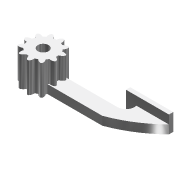
# Autodesk Inventor part: Greifer2
Saved by Autodesk Inventor 2015 (Build 190159000, 159)
## iProperties
Created: 2015-02-07
Part Number: Greifer2
Material: ABS-Kunststoff
Document SubType Name: Modeling
Designer: Luki
Density: 1.06 g/cm^3
Appearance: Chrom - poliert
Author: Luki
Autodesk Inventor part; units mm, degrees
ref_plane "YZ Plane" through (0, 0, 0) normal (1, 0, 0) x (0, 1, 0)
ref_plane "XZ Plane" through (0, 0, 0) normal (0, 1, 0) x (-1, 0, 0)
ref_plane "XY Plane" through (0, 0, 0) normal (0, 0, 1) x (1, 0, 0)
sketch "Skizze1" plane through (0, 0, 0) normal (0, 0, 1) x (1, 0, 0)
  circle A0 centre (0, 0) radius 7.5
  circle A1 centre (0, 0) radius 2
  circle A2 centre (0, 0) radius 6.5
  circle A3 centre (0, 0) radius 8.5
  line L0 (0, 11.9067) -> (0, -11.9011) projected
  line L1 (-11.9, 0) -> (11.9, 0) projected
  line L2 (0, 0) -> (2.2933, 8.1848)
  line L3 (0, 0) -> (4.4165, 7.2626)
  arc A4 (0, 7.5) -> (-0.3402, 6.4911) centre (2.4347, 6.1172) ccw
  arc A5 (0.8885, 8.4534) -> (0, 7.5) centre (2.4473, 6.1101) ccw
  arc A6 (2.0235, 7.2219) -> (1.4252, 8.3797) centre (-0.708, 6.5438) ccw
  arc A7 (2.0788, 6.1586) -> (2.0235, 7.2219) centre (-0.694, 6.5473) ccw
  line L4 (0, 0) -> (-0.3402, 6.4911)
  line L5 (0, 0) -> (2.0788, 6.1586)
  line L6 (0.8885, 8.4534) -> (0, 0)
  line L7 (0, 0) -> (1.4252, 8.3797)
  arc A8 (0, 7.5) -> (-0.3402, 6.4911) centre (2.4347, 6.1172) ccw
  arc A9 (0.8885, 8.4534) -> (0, 7.5) centre (2.4473, 6.1101) ccw
  arc A10 (2.0235, 7.2219) -> (1.4252, 8.3797) centre (-0.708, 6.5438) ccw
  arc A11 (2.0788, 6.1586) -> (2.0235, 7.2219) centre (-0.694, 6.5473) ccw
  arc A12 (2.0788, 6.1586) -> (-0.3402, 6.4911) centre (0, 0) ccw
  dimension "d0" = 15
  dimension "d1" = 4
  dimension "d2" = 1
  dimension "d3" = 1
  dimension "d4" = 15.652
  dimension "d5" = 15.652
  dimension "d6" = 3
  dimension "d7" = 3
  dimension "d9" = 6
  dimension "d10" = 6
  dimension "d11" = 2.8
  dimension "d12" = 2.8
  constraints: 26 point on circle, 13 centre point, 12 end point, 7 tangent, 4 coincident, 3 concentric, 2 point on line
  measures "d0" diameter of A0
  measures "d1" diameter of A1
  measures "d2" radial gap between concentric circles of A0 A2
  measures "d3" radial gap between concentric circles of A3 A0
  measures "d4" angle of L0 L2
  measures "d5" angle of L2 L3
  measures "d6" angle of L0 L4
  measures "d7" angle of L2 L5
  measures "d9" angle of L0 L6
  measures "d10" angle of L2 L7
  measures "d11" radius of A4
  measures "d12" radius of A7
extrude "Extrusion1" add sketch "Skizze1" along normal blind 14 contours L2 A2 L7 A0 | A7 A2 L2 | A0 L7 A6 | L7 A2 L6 A0 | A0 L6 A3 L7 | L2 A1 L7 A2 | A5 L6 A0 | A0 L6 A2 L0 | L0 A2 A4 | L4 A1 L0 | L7 A1 L2 | L0 A1 L6 | L6 A1 L7 | L7 A1 L6 A2 | L0 A1 L4 A2 | A2 L6 A1 L0
pattern_circular "Runde Anordnung1" count 11 over 360 about axis through (0, 0, -10) along (0, 0, 1) of "Extrusion1"
sketch "Skizze2" plane through (0, 0, 14) normal (0, 0, 1) x (0.8118, 0.5839, 0)
  arc A0 (5.6575, 6.3437) -> (4.3795, 6.0885) centre (5.5546, 3.5312) ccw projected
  arc A1 (6.0501, 5.9705) -> (5.6575, 6.3437) centre (0, 0) ccw projected
  arc A2 (5.8597, 4.6812) -> (6.0501, 5.9705) centre (3.2463, 5.7257) ccw projected
  arc A3 (5.2838, 3.7857) -> (5.8597, 4.6812) centre (3.2597, 5.7204) ccw projected
  arc A4 (5.2838, 3.7857) -> (5.0784, 4.057) centre (0, 0) ccw projected
  line L0 (5.0784, 4.057) -> (0, 0) projected
  line L1 (0, 0) -> (5.9126, 2.7002) projected
  arc A5 (6.9759, 2.7543) -> (5.9126, 2.7002) centre (6.5839, -0.0181) ccw projected
  arc A6 (8.1891, 2.278) -> (6.9759, 2.7543) centre (6.5819, -0.0324) ccw projected
  arc A7 (8.3175, 1.7518) -> (8.1891, 2.278) centre (0, 0) ccw projected
  arc A8 (7.4604, 0.7701) -> (8.3175, 1.7518) centre (5.8266, 3.0617) ccw projected
  arc A9 (6.4917, 0.3281) -> (7.4604, 0.7701) centre (5.8349, 3.05) ccw projected
  arc A10 (6.4917, 0.3281) -> (6.4656, 0.6674) centre (0, 0) ccw projected
  line L2 (6.4656, 0.6674) -> (0, 0) projected
  line L3 (0, 0) -> (-4.9124, -4.2566) projected
  arc A11 (-5.9174, -4.6081) -> (-4.9124, -4.2566) centre (-6.3224, -1.8375) ccw projected
  arc A12 (-7.2155, -4.4929) -> (-5.9174, -4.6081) centre (-6.3244, -1.8233) ccw projected
  arc A13 (-7.4871, -4.0241) -> (-7.2155, -4.4929) centre (0, 0) ccw projected
  arc A14 (-6.9412, -2.8407) -> (-7.4871, -4.0241) centre (-4.728, -4.5792) ccw projected
  arc A15 (-6.1363, -2.1437) -> (-6.9412, -2.8407) centre (-4.7393, -4.5703) ccw projected
  arc A16 (-6.1363, -2.1437) -> (-6.0157, -2.4619) centre (0, 0) ccw projected
  line L4 (-6.0157, -2.4619) -> (0, 0) projected
  line L5 (-6.3918, 1.1812) -> (0, 0) projected
  arc A17 (-6.3212, 1.5141) -> (-6.3918, 1.1812) centre (0, 0) ccw projected
  arc A18 (-6.3212, 1.5141) -> (-7.3751, 1.363) centre (-6.4578, -1.2825) ccw projected
  arc A19 (-7.3751, 1.363) -> (-8.4741, 0.6625) centre (-6.4531, -1.2961) ccw projected
  arc A20 (-8.4741, 0.6625) -> (-8.4991, 0.1214) centre (0, 0) ccw projected
  arc A21 (-8.4991, 0.1214) -> (-7.4693, -0.6774) centre (-6.3062, 1.8854) ccw projected
  arc A22 (-7.4693, -0.6774) -> (-6.4338, -0.925) centre (-6.3121, 1.8723) ccw projected
  line L6 (0, 0) -> (-6.4338, -0.925) projected
  line L7 (-3.7297, -5.3235) -> (0, 0) projected
  arc A23 (-4.0032, -5.121) -> (-3.7297, -5.3235) centre (0, 0) ccw projected
  arc A24 (-4.0032, -5.121) -> (-4.3035, -6.1425) centre (-1.516, -6.4071) ccw projected
  arc A25 (-4.3035, -6.1425) -> (-4.1229, -7.4331) centre (-1.5017, -6.4084) ccw projected
  arc A26 (-4.1229, -7.4331) -> (-3.6411, -7.6807) centre (0, 0) ccw projected
  arc A27 (-3.6411, -7.6807) -> (-2.4867, -7.0757) centre (-4.3347, -4.9531) ccw projected
  arc A28 (-2.4867, -7.0757) -> (-1.8313, -6.2367) centre (-4.3253, -4.9639) ccw projected
  line L8 (0, 0) -> (-1.8313, -6.2367) projected
  arc A29 (4.3795, 6.0885) -> (3.5142, 5.4681) centre (5.5486, 3.5443) ccw projected
  line L9 (0, 0) -> (3.5142, 5.4681) projected
  line L10 (-4.7385, 4.4494) -> (0, 0) projected
  line L11 (0, 0) -> (1.8313, -6.2367) projected
  arc A30 (1.7335, -7.2969) -> (1.8313, -6.2367) centre (-0.9549, -6.5144) ccw projected
  arc A31 (1.0894, -8.4299) -> (1.7335, -7.2969) centre (-0.9688, -6.5103) ccw projected
  arc A32 (0.5502, -8.4822) -> (1.0894, -8.4299) centre (0, 0) ccw projected
  arc A33 (-0.2995, -7.494) -> (0.5502, -8.4822) centre (2.2013, -6.203) ccw projected
  arc A34 (-0.5991, -6.4723) -> (-0.2995, -7.494) centre (2.1885, -6.2096) ccw projected
  arc A35 (-0.5991, -6.4723) -> (-0.2596, -6.4948) centre (0, 0) ccw projected
  line L12 (-0.2596, -6.4948) -> (0, 0) projected
  line L13 (-1.5808, 6.3049) -> (0, 0) projected
  arc A36 (-1.2486, 6.3789) -> (-1.5808, 6.3049) centre (0, 0) ccw projected
  arc A37 (-1.2486, 6.3789) -> (-1.824, 7.2748) centre (-3.8493, 5.3415) ccw projected
  arc A38 (-1.824, 7.2748) -> (-2.9176, 7.9836) centre (-3.8597, 5.3315) ccw projected
  arc A39 (-2.9176, 7.9836) -> (-3.4203, 7.7815) centre (0, 0) ccw projected
  arc A40 (-3.4203, 7.7815) -> (-3.719, 6.513) centre (-0.9047, 6.5195) ccw projected
  arc A41 (-3.719, 6.513) -> (-3.5142, 5.4681) centre (-0.919, 6.5195) ccw projected
  line L14 (0, 0) -> (-3.5142, 5.4681) projected
  line L15 (3.293, -5.6041) -> (0, 0) projected
  arc A42 (2.9952, -5.7688) -> (3.293, -5.6041) centre (0, 0) ccw projected
  arc A43 (2.9952, -5.7688) -> (3.7996, -6.4663) centre (5.1983, -4.0406) ccw projected
  arc A44 (3.7996, -6.4663) -> (5.0487, -6.8382) centre (5.2055, -4.0282) ccw projected
  arc A45 (5.0487, -6.8382) -> (5.474, -6.5027) centre (0, 0) ccw projected
  arc A46 (5.474, -6.5027) -> (5.4033, -5.2014) centre (2.7048, -6.0006) ccw projected
  arc A47 (5.4033, -5.2014) -> (4.9124, -4.2566) centre (2.7186, -5.9965) ccw projected
  line L16 (0, 0) -> (4.9124, -4.2566) projected
  arc A48 (-4.4991, 4.6913) -> (-4.7385, 4.4494) centre (0, 0) ccw projected
  arc A49 (-4.4991, 4.6913) -> (-5.4675, 5.1339) centre (-6.1261, 2.4124) ccw projected
  arc A50 (-5.4675, 5.1339) -> (-6.7707, 5.1388) centre (-6.1295, 2.3984) ccw projected
  arc A51 (-6.7707, 5.1388) -> (-7.0843, 4.6971) centre (0, 0) ccw projected
  arc A52 (-7.0843, 4.6971) -> (-6.6498, 3.4684) centre (-4.2858, 4.9955) ccw projected
  arc A53 (-6.6498, 3.4684) -> (-5.9126, 2.7002) centre (-4.2979, 4.9877) ccw projected
  line L17 (0, 0) -> (-5.9126, 2.7002) projected
  line L18 (2.0788, 6.1586) -> (0, 0) projected
  line L19 (0, 0) -> (6.4338, -0.925) projected
  arc A54 (7.3576, -1.4544) -> (6.4338, -0.925) centre (5.529, -3.5748) ccw projected
  arc A55 (8.1207, -2.5109) -> (7.3576, -1.4544) centre (5.5196, -3.5857) ccw projected
  arc A56 (7.9442, -3.0231) -> (8.1207, -2.5109) centre (0, 0) ccw projected
  arc A57 (6.6924, -3.3856) -> (7.9442, -3.0231) centre (6.5569, -0.5744) ccw projected
  arc A58 (5.6386, -3.2337) -> (6.6924, -3.3856) centre (6.5576, -0.5888) ccw projected
  arc A59 (5.6386, -3.2337) -> (5.8001, -2.9341) centre (0, 0) ccw projected
  line L20 (5.8001, -2.9341) -> (0, 0) projected
  arc A60 (2.3983, 6.0414) -> (2.0788, 6.1586) centre (0, 0) ccw projected
  arc A61 (2.3983, 6.0414) -> (2.3987, 7.1061) centre (-0.3504, 6.5746) ccw projected
  arc A62 (2.3987, 7.1061) -> (1.8618, 8.2936) centre (-0.3646, 6.5719) ccw projected
  arc A63 (1.8618, 8.2936) -> (1.3297, 8.3954) centre (0, 0) ccw projected
  arc A64 (1.3297, 8.3954) -> (0.3925, 7.4897) centre (2.7637, 5.9737) ccw projected
  arc A65 (0.3925, 7.4897) -> (0, 6.5) centre (2.7516, 5.9814) ccw projected
  line L21 (0, 0) -> (0, 6.5) projected
  circle A66 centre (0, 0) radius 6.5
  constraints: 1 centre point, 1 coincident
extrude "Extrusion2" add sketch "Skizze2" against normal blind 14 contours A66 L0 L9 | L9 L18 A60 A66 | L0 A4 A66 L1 | L1 A66 L2 | L7 A23 A66 L3 | L3 A66 L4 | L6 A66 L5 | L4 A16 A66 L6 | L8 A66 L7 | L12 A35 A66 L8 | L17 A66 L10 | L15 A42 A66 L11 | L11 A66 L12 | L14 A66 L13 | L10 A48 A66 L14 | L16 A66 L15 | L20 A59 A66 L16 | L5 A17 A66 L17 | L21 A66 L18 | L2 A10 A66 L19 | L19 A66 L20 | L13 A36 A66 L21
sketch "Skizze3" plane through (0, 0, 0) normal (0, 0, -1) x (-1, 0, 0)
  line L0 (0, -19.7919) -> (0, 59.2516) projected
  line L1 (-62.4254, 0) -> (20.3695, 0) projected
  arc A0 (0, 7.5) -> (-0.8885, 8.4534) centre (-2.4473, 6.1101) ccw projected
  arc A1 (0.3402, 6.4911) -> (0, 7.5) centre (-2.4347, 6.1172) ccw projected
  arc A2 (1.5808, 6.3049) -> (0.3402, 6.4911) centre (0, 0) ccw projected
  arc A3 (2.2022, 7.1694) -> (1.5808, 6.3049) centre (4.1236, 5.1327) ccw projected
  arc A4 (3.3315, 7.8199) -> (2.2022, 7.1694) centre (4.1335, 5.1222) ccw projected
  arc A5 (3.8228, 7.5918) -> (3.3315, 7.8199) centre (0, 0) ccw projected
  arc A6 (4.0548, 6.3094) -> (3.8228, 7.5918) centre (1.2446, 6.4633) ccw projected
  arc A7 (3.7955, 5.2767) -> (4.0548, 6.3094) centre (1.259, 6.4625) ccw projected
  arc A8 (4.7385, 4.4494) -> (3.7955, 5.2767) centre (0, 0) ccw projected
  arc A9 (5.7287, 4.8407) -> (4.7385, 4.4494) centre (6.2439, 2.0885) ccw projected
  arc A10 (7.0304, 4.7774) -> (5.7287, 4.8407) centre (6.2466, 2.0744) ccw projected
  arc A11 (7.3204, 4.3199) -> (7.0304, 4.7774) centre (0, 0) ccw projected
  arc A12 (6.8222, 3.1156) -> (7.3204, 4.3199) centre (4.5413, 4.7644) ccw projected
  arc A13 (6.0458, 2.3871) -> (6.8222, 3.1156) centre (4.553, 4.7559) ccw projected
  arc A14 (6.3918, 1.1812) -> (6.0458, 2.3871) centre (0, 0) ccw projected
  arc A15 (7.4363, 0.9751) -> (6.3918, 1.1812) centre (6.3819, -1.6188) ccw projected
  arc A16 (8.4972, 0.2181) -> (7.4363, 0.9751) centre (6.3765, -1.6321) ccw projected
  arc A17 (8.4938, -0.3236) -> (8.4972, 0.2181) centre (0, 0) ccw projected
  arc A18 (7.4237, -1.0674) -> (8.4938, -0.3236) centre (6.3962, 1.5528) ccw projected
  arc A19 (6.3766, -1.2605) -> (7.4237, -1.0674) centre (6.4015, 1.5394) ccw projected
  arc A20 (6.0157, -2.4619) -> (6.3766, -1.2605) centre (0, 0) ccw projected
  arc A21 (6.783, -3.2001) -> (6.0157, -2.4619) centre (4.4936, -4.8121) ccw projected
  arc A22 (7.2662, -4.4104) -> (6.783, -3.2001) centre (4.4818, -4.8204) ccw projected
  arc A23 (6.9705, -4.8643) -> (7.2662, -4.4104) centre (0, 0) ccw projected
  arc A24 (5.6681, -4.9115) -> (6.9705, -4.8643) centre (6.2204, -2.1518) ccw projected
  arc A25 (4.6829, -4.5079) -> (5.6681, -4.9115) centre (6.2175, -2.1659) ccw projected
  arc A26 (3.7297, -5.3235) -> (4.6829, -4.5079) centre (0, 0) ccw projected
  arc A27 (3.9761, -6.3593) -> (3.7297, -5.3235) centre (1.1787, -6.4776) ccw projected
  arc A28 (3.7283, -7.6387) -> (3.9761, -6.3593) centre (1.1643, -6.4782) ccw projected
  arc A29 (3.2341, -7.8607) -> (3.7283, -7.6387) centre (0, 0) ccw projected
  arc A30 (2.113, -7.1962) -> (3.2341, -7.8607) centre (4.0696, -5.1732) ccw projected
  arc A31 (1.5023, -6.324) -> (2.113, -7.1962) centre (4.0595, -5.1835) ccw projected
  arc A32 (0.2596, -6.4948) -> (1.5023, -6.324) centre (0, 0) ccw projected
  arc A33 (-0.0931, -7.4994) -> (0.2596, -6.4948) centre (-2.5105, -6.0865) ccw projected
  arc A34 (-0.9934, -8.4418) -> (-0.0931, -7.4994) centre (-2.5229, -6.0793) ccw projected
  arc A35 (-1.5291, -8.3613) -> (-0.9934, -8.4418) centre (0, 0) ccw projected
  arc A36 (-2.113, -7.1962) -> (-1.5291, -8.3613) centre (0.6267, -6.5521) ccw projected
  arc A37 (-2.1552, -6.1323) -> (-2.113, -7.1962) centre (0.6127, -6.5554) ccw projected
  arc A38 (-3.293, -5.6041) -> (-2.1552, -6.1323) centre (0, 0) ccw projected
  arc A39 (-4.1328, -6.2586) -> (-3.293, -5.6041) centre (-5.4026, -3.763) ccw projected
  arc A40 (-5.3996, -6.5646) -> (-4.1328, -6.2586) centre (-5.4091, -3.7502) ccw projected
  arc A41 (-5.8068, -6.2073) -> (-5.3996, -6.5646) centre (0, 0) ccw projected
  arc A42 (-5.6681, -4.9115) -> (-5.8068, -6.2073) centre (-3.0151, -5.8508) ccw projected
  arc A43 (-5.1284, -3.9937) -> (-5.6681, -4.9115) centre (-3.0287, -5.846) ccw projected
  arc A44 (-5.8001, -2.9341) -> (-5.1284, -3.9937) centre (0, 0) ccw projected
  arc A45 (-6.8604, -3.0307) -> (-5.8001, -2.9341) centre (-6.5794, -0.2448) ccw projected
  arc A46 (-8.0916, -2.6032) -> (-6.8604, -3.0307) centre (-6.578, -0.2305) ccw projected
  arc A47 (-8.2409, -2.0825) -> (-8.0916, -2.6032) centre (0, 0) ccw projected
  arc A48 (-7.4237, -1.0674) -> (-8.2409, -2.0825) centre (-5.6997, -3.2919) ccw projected
  arc A49 (-6.4734, -0.5871) -> (-7.4237, -1.0674) centre (-5.7085, -3.2805) ccw projected
  arc A50 (-6.4656, 0.6674) -> (-6.4734, -0.5871) centre (0, 0) ccw projected
  arc A51 (-7.4098, 1.1595) -> (-6.4656, 0.6674) centre (-5.6673, 3.3512) ccw projected
  arc A52 (-8.2145, 2.1847) -> (-7.4098, 1.1595) centre (-5.6583, 3.3624) ccw projected
  arc A53 (-8.0586, 2.7035) -> (-8.2145, 2.1847) centre (0, 0) ccw projected
  arc A54 (-6.8222, 3.1156) -> (-8.0586, 2.7035) centre (-6.5746, 0.3121) ccw projected
  arc A55 (-5.7632, 3.0059) -> (-6.8222, 3.1156) centre (-6.5759, 0.3265) ccw projected
  arc A56 (-5.0784, 4.057) -> (-5.7632, 3.0059) centre (0, 0) ccw projected
  arc A57 (-5.6067, 4.9815) -> (-5.0784, 4.057) centre (-2.9559, 5.8832) ccw projected
  arc A58 (-5.7293, 6.2789) -> (-5.6067, 4.9815) centre (-2.9422, 5.8878) ccw projected
  arc A59 (-5.3177, 6.6311) -> (-5.7293, 6.2789) centre (0, 0) ccw projected
  arc A60 (-4.0548, 6.3094) -> (-5.3177, 6.6311) centre (-5.3622, 3.8171) ccw projected
  arc A61 (-3.2232, 5.6446) -> (-4.0548, 6.3094) centre (-5.3555, 3.8298) ccw projected
  arc A62 (-2.0788, 6.1586) -> (-3.2232, 5.6446) centre (0, 0) ccw projected
  arc A63 (-2.0235, 7.2219) -> (-2.0788, 6.1586) centre (0.694, 6.5473) ccw projected
  arc A64 (-1.4252, 8.3797) -> (-2.0235, 7.2219) centre (0.708, 6.5438) ccw projected
  arc A65 (-0.8885, 8.4534) -> (-1.4252, 8.3797) centre (0, 0) ccw projected
  circle A66 centre (0, 0) radius 3.5
  line L2 (-50, 10.5) -> (-30, 10.5)
  line L3 (-30, 10.5) -> (-30, 8.5)
  line L4 (-30, 8.5) -> (-50, 8.5)
  line L5 (-50, 8.5) -> (-50, 10.5)
  circle A67 centre (0, 0) radius 8.5
  arc A68 (-5.3177, 6.6311) -> (-5.7293, 6.2789) centre (0, 0) ccw projected
  line L6 (0, -3.5) -> (-31, -3.5)
  line L7 (-31, -3.5) -> (-31, 3.5)
  line L8 (-31, 3.5) -> (0, 3.5)
  line L9 (0, 3.5) -> (0, -3.5)
  arc A69 (-34.873, 8.5) -> (-31, 3.5) centre (-31, 7.5) ccw
  arc A70 (-50, 8.5) -> (-31, -3.5) centre (-12.2955, 47.1571) ccw
  dimension "d24" = 7
  dimension "d20" = 2
  dimension "d21" = 0
  dimension "d22" = 50
  dimension "d23" = 30
  dimension "d25" = 54
  dimension "d26" = 7
  dimension "d27" = 4
  dimension "d28" = 31
  constraints: 16 end point, 4 parallel, 4 point on circle, 3 centre point, 2 coincident, 2 horizontal, 2 perpendicular, 2 point on line, 2 tangent, 1 vertical alignment, 2 other
  measures "d20" distance between parallel lines of L2 L4
  measures "d21" distance edge to line of A67 L4
  measures "d22" distance between parallel lines of L0 L5
  measures "d23" distance between parallel lines of L0 L3
  measures "d25" radius of A70
  measures "d26" distance from line of L8 L6.end
  measures "d27" radius of A69
  measures "d28" distance between parallel lines of L0 L7
extrude "Extrusion3" add sketch "Skizze3" against normal blind 4 contours A66 L1 L0 | L0 L1 A66 | A66 L1 A50 A51 A52 A53 A54 A55 A56 L8 | L1 A66 L0 | L0 A66 L1 | A66 L6 A44 A45 A46 A47 A48 A49 A50 L1 | A56 A55 A54 A67 L8 | A50 A49 A48 A67 L1 | L1 A67 A52 A51 A50 | A67 A53 L1 L7 L8 | L6 A67 A46 A45 A44 | A67 A47 L6 L7 L1 | L7 L1 A70 L4 A69 | L7 A70 L1 | L4 L5 L2 L3
sketch "Skizze4" plane through (0, 0, 14) normal (0, 0, 1) x (1, 0, 0)
  circle A0 centre (0, 0) radius 2.5
  dimension "d31" = 5
  constraints: 1 centre point, 1 coincident
  measures "d31" diameter of A0
extrude "Extrusion4" cut sketch "Skizze4" against normal through all
sketch "Skizze5" plane through (0, 0, 4) normal (0, 0, 1) x (1, 0, 0)
  line L0 (30, 8.5) -> (50, 8.5)
  line L1 (50, 8.5) -> (50, 10.5)
  line L2 (50, 10.5) -> (30, 10.5)
  line L3 (30, 10.5) -> (30, 8.5)
  point P0 (0, 0)
  constraints: 8 end point, 2 parallel, 1 horizontal, 1 perpendicular
extrude "Extrusion5" add sketch "Skizze5" along normal blind 4
equation "\"d5\" = d4"
equation "\"d7\" = d6"
equation "\"d12\" = d11"
